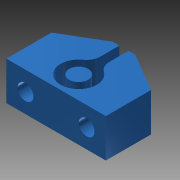
# Autodesk Inventor part: XCarriageBeltClipRound
Saved by Autodesk Inventor 2016 (Build 200138000, 138)
## iProperties
Category: Print
Created: 2014-12-16
Part Number: XCarriageBeltClipRound
Material: Generic
Document SubType Name: Modeling
Designer: Jack
Density: 1 g/cm^3
Appearance: Cyan
Mass: 1.62871 g
Surface Area: 17.7624 cm^2
Volume: 1.62871 cm^3
Author: Jack
Title: X Carriage Belt Clip
Autodesk Inventor part; units mm, degrees
ref_plane "YZ Plane" through (0, 0, 0) normal (1, 0, 0) x (0, 1, 0)
ref_plane "XZ Plane" through (0, 0, 0) normal (0, 1, 0) x (-1, 0, 0)
ref_plane "XY Plane" through (0, 0, 0) normal (0, 0, 1) x (1, 0, 0)
sketch "Sketch1" plane through (0, 0, 0) normal (0, 0, 1) x (1, 0, 0)
  line L0 (0, 0) -> (22, 0)
  line L1 (22, 0) -> (22, 10)
  line L2 (0, 0) -> (0, 10)
  line L3 (8.5, 15) -> (13.5, 15)
  line L4 (13.5, 15) -> (22, 10)
  line L5 (8.5, 15) -> (0, 10)
  dimension "d0" = 22
  dimension "d1" = 10
  dimension "d2" = 5
  dimension "d3" = 5
  constraints: 12 end point, 2 horizontal, 1 equal length, 1 horizontal alignment, 1 perpendicular, 1 vertical
  measures "d0" distance of L0.start L0.end
  measures "d1" distance of L0.end L1.end
  measures "d2" distance of L3.start L3.end
  measures "d3" distance from line of L1.end L3
extrude "Extrusion1" add sketch "Sketch1" along normal blind 8.5
sketch "Sketch2" plane through (0, 0, 8.5) normal (0, 0, 1) x (1, 0, 0)
  line L0 (0, 0) -> (22, 0) projected
  line L1 (22, 0) -> (22, 10) projected
  line L2 (13.5, 15) -> (8.5, 15) projected
  arc A0 (10, 8.873) -> (12, 8.873) centre (11, 5) ccw
  circle A1 centre (11, 5) radius 2.1
  line L3 (10, 15) -> (10, 8.873)
  line L4 (12, 8.873) -> (12, 15)
  dimension "d6" = 8
  dimension "d7" = 4.2
  dimension "d8" = 5
  dimension "d9" = 11
  dimension "d10" = 2
  dimension "d11" = 1
  constraints: 4 end point, 2 centre point, 2 point on circle, 2 point on line, 1 coincident, 1 perpendicular, 1 vertical
  measures "d6" diameter of A0
  measures "d7" diameter of A1
  measures "d8" distance from line of L0 A0.centre
  measures "d9" distance from line of L1 A0.centre
  measures "d10" distance between parallel lines of L3 L4
  measures "d11" distance from line of A0.centre L4
extrude "Extrusion2" cut sketch "Sketch2" against normal blind 7.5
fillet "Fillet1" radius 3 2 edges at (12, 8.873, 4.75) (10, 8.873, 4.75)
sketch "Sketch3" plane through (8.5, 15, 0) normal (0, 1, 0) x (1, 0, 0)
  line L0 (13.5, 0) -> (5, 0) projected
  line L1 (5, 0) -> (5, -8.5) projected
  line L2 (13.5, -8.5) -> (5, -8.5) projected
  line L3 (13.5, 0) -> (13.5, -8.5) projected
  line L4 (0, 0) -> (-8.5, 0) projected
  line L5 (-8.5, 0) -> (-8.5, -8.5) projected
  line L6 (0, -8.5) -> (-8.5, -8.5) projected
  line L7 (0, 0) -> (0, -8.5) projected
  point P0 (9.25, -4.25)
  point P1 (-4.25, -4.25)
  dimension "d15" = 13.5
  dimension "d16" = 4.25
  dimension "d17" = 4.25
  constraints: 1 horizontal alignment
  measures "d15" distance of point (9.25, -4.25) point (-4.25, -4.25)
  measures "d16" distance from line of L5 point (-4.25, -4.25)
  measures "d17" distance from line of L6 point (-4.25, -4.25)
hole "Hole1" at (17.75, 15, 4.25) at (4.25, 15, 4.25) direction (0, -1, 0) diameter 3.5 end through all counterbore diameter 8 counterbore depth 5
body "Solid1"
